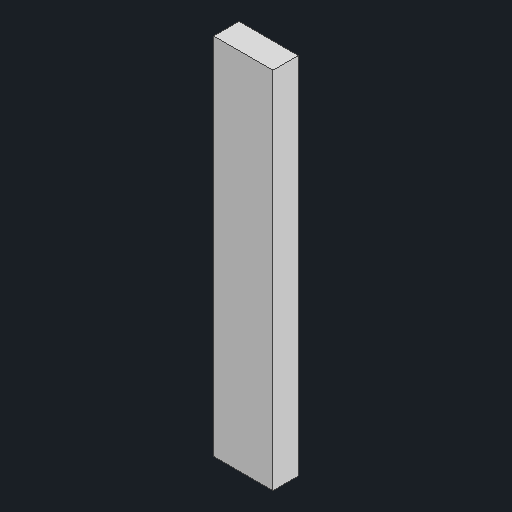
# Autodesk Inventor part: 2x4x21.5
Saved by Autodesk Inventor 2026 (Build 300175000, 175)
## iProperties
Created: 2024-09-20
Part Number: 2x4x21.5
Material: Generic
Document SubType Name: Modeling
Designer: User
Density: 1 g/cm^3
Appearance: Default
Author: User
Autodesk Inventor part; units mm, degrees
ref_plane "YZ Plane" through (0, 0, 0) normal (1, 0, 0) x (0, 1, 0)
ref_plane "XZ Plane" through (0, 0, 0) normal (0, 1, 0) x (-1, 0, 0)
ref_plane "XY Plane" through (0, 0, 0) normal (0, 0, 1) x (1, 0, 0)
sketch "Sketch1" plane through (0, 0, 0) normal (0, 0, 1) x (1, 0, 0)
  line L0 (-848.7411, -635) -> (-437.8392, -635) projected
  line L1 (0, -88.9) -> (-1697.4822, -88.9) projected
  line L2 (-437.8392, -88.9) -> (-526.7392, -88.9)
  line L3 (-1697.4822, -635) -> (-848.7411, -635) projected
  line L4 (-848.7411, -635) -> (-848.7411, -88.9)
  line L5 (-937.6411, -635) -> (-937.6411, -88.9)
  point P0 (0, 0)
  dimension "d3" = 88.9
  constraints: 6 end point, 4 point on line, 1 midpoint, 1 perpendicular
  measures "d3" distance between parallel lines of L5 L4
extrude "Extrusion1" add sketch "Sketch1" against normal blind 38.1
body "Solid1"
